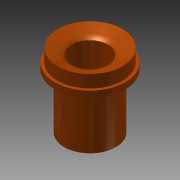
# Autodesk Inventor part: Phenolic
Saved by Autodesk Inventor 2015 (Build 190159000, 159)
## iProperties
Created: 2016-01-09
Part Number: Phenolic
Material: Phenolic Resin
Document SubType Name: Modeling
Designer: Jared
Density: 1.38 g/cm^3
Appearance: Smooth - Light Orange
Author: Jared
Autodesk Inventor part; units mm, degrees
ref_plane "YZ Plane" through (0, 0, 0) normal (1, 0, 0) x (0, 1, 0)
ref_plane "XZ Plane" through (0, 0, 0) normal (0, 1, 0) x (-1, 0, 0)
ref_plane "XY Plane" through (0, 0, 0) normal (0, 0, 1) x (1, 0, 0)
sketch "Sketch1" plane through (0, 0, 0) normal (0, 0, 1) x (1, 0, 0)
  arc A0 (-19.4827, -3.287) -> (-19.05, 0) centre (-31.75, 0) ccw
  line L0 (-19.4827, -3.287) -> (-58.7375, -149.7878)
  line L1 (-65.8876, 46.8376) -> (-65.8876, 21.4376)
  line L2 (-65.8876, 21.4376) -> (-71.4375, 21.4376)
  line L3 (-44.45, 34.1376) -> (-36.591, 34.1376)
  line L4 (-44.45, 34.1376) -> (-37.3992, -46.4536)
  line L5 (-44.45, 34.1376) -> (0, 34.1376) construction
  line L6 (-37.3992, -46.4536) -> (-31.0492, -46.4536)
  line L7 (-71.4375, 21.4376) -> (-71.4375, 8.7376)
  line L8 (-71.4375, 8.7376) -> (-58.7375, 8.7376)
  line L9 (-58.7375, 8.7376) -> (-52.3875, 8.7376)
  line L10 (-52.3875, 8.7376) -> (-52.3875, -102.3907)
  line L11 (-71.4375, 8.7376) -> (-71.4375, -0.7874)
  line L12 (-71.4375, 8.7376) -> (-61.9125, 8.7376) construction
  line L13 (-71.4375, -0.7874) -> (-58.7375, -0.7874)
  line L14 (-58.7375, -0.7874) -> (-58.7375, -51.5874)
  line L15 (-58.7375, -51.5874) -> (-71.4375, -51.5874)
  line L16 (-71.4375, -0.7874) -> (-65.0875, -0.7874)
  line L17 (-65.0875, -0.7874) -> (-65.0875, -6.731)
  line L18 (-65.0875, -6.731) -> (-71.4375, -6.731)
  line L19 (-71.4375, 21.4376) -> (-71.4375, -0.7874)
  line L20 (-71.4375, -6.731) -> (-71.4375, -51.5874)
  line L21 (-58.7375, -51.5874) -> (-58.7375, -126.0892)
  line L22 (-58.7375, -51.5874) -> (0, -51.5874) construction
  line L23 (-46.0375, -102.3907) -> (-52.3875, -102.3907)
  line L24 (-65.0875, -51.5907) -> (-58.7375, -51.5907)
  line L25 (-58.7375, -149.7878) -> (-61.9125, -161.637)
  line L26 (-58.7375, -149.7878) -> (-34.203, -149.7878) construction
  line L27 (-65.0875, -161.637) -> (-61.9125, -161.637)
  line L28 (-58.7375, -126.0892) -> (-52.3875, -126.0892)
  line L29 (0, 34.1376) -> (0, 0)
  line L30 (-65.0875, -100.6892) -> (-65.0875, -161.637)
  line L31 (-58.7375, -51.5907) -> (-61.9125, -51.5907)
  line L32 (-65.0875, -100.6892) -> (-58.7375, -100.6892)
  line L33 (-65.8876, 46.8376) -> (-18.3062, 46.8376) construction
  arc A1 (-19.05, 0) -> (-45.9916, 39.2002) centre (-61.0391, 0) ccw
  line L34 (-65.8876, 46.8376) -> (-14.7047, 46.8376) construction
  line L35 (-65.8876, 46.8376) -> (-45.9916, 39.2002)
  dimension "d56" = 19.05
  dimension "d57" = 25.4
  dimension "d58" = 5.5499
  dimension "d59" = 65.8876
  dimension "d60" = 85
  dimension "d61" = 12.7
  dimension "d62" = 12.7
  dimension "d63" = 44.45
  dimension "d64" = 6.35
  dimension "d65" = 105
  dimension "d66" = 12.7
  dimension "d67" = 12.7
  dimension "d68" = 6.35
  dimension "d69" = 9.525
  dimension "d70" = 50.8
  dimension "d71" = 12.7
  dimension "d72" = 6.35
  dimension "d73" = 5.9436
  dimension "d74" = 6.35
  dimension "d75" = 50.8
  dimension "d76" = 6.35
  dimension "d77" = 105
  dimension "d78" = 3.175
  dimension "d79" = 6.35
  dimension "d80" = 60.9478
  dimension "d81" = 3.175
  dimension "d82" = 6.35
  dimension "d83" = 25.4
  dimension "d84" = 41.9891
  dimension "d85" = 21
  constraints: 73 end point, 15 perpendicular, 11 horizontal, 7 point on line, 5 point on circle, 4 vertical, 3 horizontal alignment, 2 centre point, 2 collinear, 2 midpoint, 2 tangent, 1 parallel, 1 vertical alignment, 1 other
  measures "d56" distance of A0.end L29.end
  measures "d57" distance of L1.start L2.start
  measures "d58" distance of L2.start L2.end
  measures "d59" distance from line of L29.end L1
  measures "d60" angle of L4 L5
  measures "d61" vertical distance of L4.start L1.start
  measures "d62" radius of A0
  measures "d63" horizontal distance of L29.end L4.start
  measures "d64" distance of L4.end L6.end
  measures "d65" angle of L6 L0
  measures "d66" distance of L2.end L12.start
  measures "d67" distance of L12.start L9.start
  measures "d68" distance of L9.start L9.end
  measures "d69" distance of L12.start L19.end
  measures "d70" distance of L13.end L22.start
  measures "d71" distance of L19.end L13.end
  measures "d72" distance of L19.end L16.end
  measures "d73" distance of L16.end L17.end
  measures "d74" distance of L10.end L23.start
  measures "d75" distance between parallel lines of L23 L24
  measures "d76" distance of L24.start L31.start
  measures "d77" angle of L25 L26
  measures "d78" distance of L25.end L27.start
  measures "d79" distance of L21.end L28.end
  measures "d80" distance of L32.start L27.start
  measures "d81" distance of L31.start L31.end
  measures "d82" distance from line of L21 L32.start
  measures "d83" distance between parallel lines of L32 L28
  measures "d84" radius of A1
  measures "d85" angle of L35 L33
revolve "Revolution1" add sketch "Sketch1" angle 360 about axis through (0, 34.1376, 0) along (0, -1, 0) contours L0 L23 L10 L9 L8 L7 L2 L1 L35 A1 L3 L4 L6
body "Solid1"
